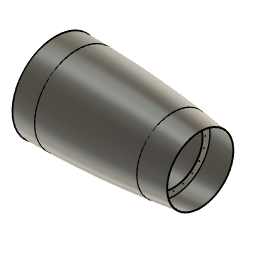
inner_body_eng_model (Autodesk Fusion 360 design; units mm, degrees)
Autodesk Fusion 360 part; units mm, degrees
sketch "Sketch1" plane through (0, 0, 0) normal (0, 1, 0) x (1, 0, 0)
  line L0 (0, 0) -> (0, -150.6845) construction
  line L1 (0, -150.6845) -> (0, -274) construction
  line L2 (0, 0) -> (910, 0) construction
  line L3 (910, 0) -> (910, -210.245) construction
  arc A0 (0, -274) -> (910, -210.245) centre (1.8405, 6225.9997) ccw
  line L4 (0, -274) -> (0, -244.36)
  line L5 (3, -271.0002) -> (3, -244.36)
  line L6 (910, -210.245) -> (910, -207.2153)
  line L7 (3, -244.36) -> (0, -244.36)
  line L8 (740, -183.31) -> (743, -183.31)
  line L9 (740, -183.31) -> (740, -228.9309)
  line L10 (743, -183.31) -> (743, -228.5871)
  line L11 (740, 0) -> (740, -228.9309) construction
  line L12 (740, -231.9504) -> (740, -347.3942) construction
  arc A1 (743, -228.5871) -> (910, -207.2153) centre (1.8405, 6225.9997) ccw
  line L13 (137, -225.43) -> (140, -225.43)
  line L14 (140, -225.43) -> (140, -269.5311)
  line L15 (137, -225.43) -> (137, -269.5942)
  line L16 (137, 0) -> (137, -269.5942) construction
  line L17 (137, -272.5949) -> (137, -306.2044) construction
  arc A2 (3, -271.0002) -> (137, -269.5942) centre (1.8405, 6225.9997) ccw
  arc A3 (140, -269.5311) -> (740, -228.9309) centre (1.8405, 6225.9997) ccw
  dimension "d1" = 274
  dimension "d2" = 910
  dimension "d3" = 210.245
  dimension "d4" = 6500
  dimension "d5" = 29.64
  dimension "d6" = 170
  dimension "d8" = 3
  dimension "d9" = 183.31
  dimension "d10" = 137
  dimension "d11" = 3
  dimension "d12" = 225.43
  constraint coincident L0.start L2.start
  constraint vertical L0
  constraint parallel L0 L1
  constraint perpendicular L0 L2
  constraint perpendicular L2 L3
  constraint coincident L1 L4.end
  constraint coincident L2 L11.start
  constraint perpendicular L2 L11
  constraint coincident L3 L6.end
  constraint concentric A0 A2
  constraint perpendicular L4 L7
  constraint coincident L8.start L11
  constraint horizontal L8
  constraint coincident L10.end A2
  constraint perpendicular L8 L10
  constraint coincident A0 L12.start
  constraint collinear L11 L12
  constraint concentric A1 A2
  constraint coincident L2 L16.start
  constraint perpendicular L2 L16
  constraint coincident L13.start L16
  constraint perpendicular L13 L16
  constraint perpendicular L13 L14
  constraint coincident A0 L17.start
  constraint collinear L16 L17
  constraint coincident L14.end A2
  constraint concentric A2 A3
  measures "d1" distance of L0.start L1.end
  measures "d2" distance of L0.start L2.end
  measures "d3" distance of L2.end L3.end
  measures "d4" radius of A0
  measures "d5" distance of L1.end L4.end
  measures "d6" distance of L3 L11
  measures "d8" distance of L8.start L8.end
  measures "d9" distance of L2 L8
  measures "d10" distance of L1 L16
  measures "d11" distance of L13.start L13.end
  measures "d12" distance of L2 L13
revolve "Revolve1" add sketch "Sketch1" angle 360 about axis through (0, 0, 0) along (1, 0, 0)
sketch "Sketch2" plane through (0, 0, 0) normal (-1, 0, 0) x (0, -1, 0)
  circle A0 centre (0, 0) radius 274
  circle A1 centre (0, 0) radius 244.36
  line L0 (0, 0) -> (0, 383.8216) construction
  circle A2 centre (0, 256.86) radius 2
  dimension "d14" = 4
  dimension "d15" = 256.86
  constraint coincident A0.centre A1.centre
  constraint vertical L0
  constraint coincident L0 A2.centre
  measures "d14" diameter of A2
  measures "d15" distance of A0.centre A2.centre
extrude "Extrude1" cut sketch "Sketch2" against normal blind 5 contours A2
pattern_circular "C-Pattern1" count 20 over 360 about axis through (1.75, 0, 0) along (1, 0, 0) of "Extrude1"
sketch "Sketch3" plane through (743, 0, 0) normal (1, 0, 0) x (0, 1, 0)
  circle A0 centre (0, 0) radius 183.31
  circle A1 centre (0, 0) radius 228.5871
  line L0 (0, 0) -> (0, 383.9772) construction
  circle A2 centre (0, 200) radius 2
  dimension "d20" = 4
  dimension "d21" = 200
  constraint coincident A0.centre A1.centre
  constraint vertical L0
  constraint coincident L0 A2.centre
  measures "d20" diameter of A2
  measures "d21" distance of A0.centre A2.centre
extrude "Extrude2" cut sketch "Sketch3" against normal blind 5 contours A2
pattern_circular "C-Pattern2" count 20 over 360 about axis through (1.75, 0, 0) along (1, 0, 0) of "Extrude2"
equation "d1 = ( 548 / 2 ) * 1 mm"
equation "d3 = ( 420.49 / 2 ) * 1 mm"
